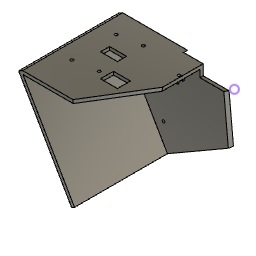
case v32 (Autodesk Fusion 360 design; units mm, degrees)
Autodesk Fusion 360 part; units mm, degrees
note: some values were not read from the file. Set by a fixed rule: which face or edge a step refers to.
ref_plane "WorkPlane2" through (0, 0, 0) normal (0, 0, 1) x (1, 0, 0) in component "Base"
sketch "top" plane through (0, 0, 0) normal (0, 0, 1) x (1, 0, 0) in component "Base"
  line L0 (-48.3808, 27.2591) -> (41.6192, 27.2591)
  line L1 (41.6192, 27.2591) -> (41.6192, -29.7409)
  line L2 (41.6192, -29.7409) -> (-48.3808, -29.7409)
  line L3 (-48.3808, -29.7409) -> (-48.3808, 27.2591)
  line L4 (5.6192, 27.2591) -> (5.6192, -29.7409) construction
  line L5 (5.6192, 27.2591) -> (41.6192, 27.2591)
  line L6 (41.6192, 27.2591) -> (41.6192, 24.2591)
  line L7 (41.6192, 24.2591) -> (5.6192, 24.2591)
  line L8 (5.6192, 24.2591) -> (5.6192, 27.2591)
  dimension "d1" = 90
  dimension "d2" = 57
  dimension "d242" = 54
  dimension "d243" = 3
  constraint horizontal L0
  constraint vertical L1
  constraint horizontal L2
  constraint vertical L3
  constraint coincident L0 L4.start
  constraint coincident L2 L4.end
  constraint perpendicular L2 L4
  constraint horizontal L5
  constraint vertical L6
  constraint horizontal L7
  constraint vertical L8
  constraint coincident L1 L6.end
  measures "d1" distance of L0.start L0.end
  measures "d2" distance of L0.start L2.end
  measures "d242" distance of L3 L4
  measures "d243" distance of L4.start L7.end
ref_plane "WorkPlane1" through (-48.3808, -1.2409, 0) normal (-0.866025, 0, -0.5) x (0, 1, 0) in component "Base"
ref_plane "WorkPlane3" through (0, 0, -1) normal (0, 0, 1) x (1, 0, 0) in component "Base"
sketch "start-dot" plane through (0, 0, -1) normal (0, 0, 1) x (1, 0, 0) in component "Base"
  line L0 (-48.3808, -29.7409) -> (-48.3808, 27.2591)
  line L1 (41.6192, -29.7409) -> (-48.3808, -29.7409)
  line L2 (-4.3808, -30.7409) -> (-14.3808, -30.7409)
  line L3 (-14.3808, -30.7409) -> (-4.3808, -30.7409)
  line L4 (-4.3808, -30.7409) -> (2.6903, -23.6698)
  line L5 (-4.3808, -30.7409) -> (3, -30.7409) construction
  point P0 (-4.3808, -30.7409)
  dimension "d25" = 44
  dimension "d32" = 10
  dimension "d33" = 10
  dimension "d117" = 45
  constraint coincident P0 L2.start
  constraint horizontal L2
  constraint parallel L3 L5
  measures "d25" distance of P0 L0
  measures "d32" distance of P0 L4.end
  measures "d33" distance of P0 L2.end
  measures "d117" angle of L4 L5
ref_plane "WorkPlane3" through (-0.8452, -27.2053, -1) normal (0.696364, -0.696364, 0.173648) x (0.707107, 0.707107, 0) in component "Base"
ref_plane "WorkPlane22" through (-4.3271, -23.7235, -1.8682) normal (0.696364, -0.696364, 0.173648) x (0.707107, 0.707107, 0) in component "Base"
sketch "table-cut" plane through (-48.3808, -1.2409, 0) normal (-0.866025, 0, -0.5) x (0, 1, 0) in component "Base"
  line L0 (-250, -250) -> (250, -250)
  line L1 (250, -250) -> (250, 250)
  line L2 (250, 250) -> (-250, 250)
  line L3 (-250, 250) -> (-250, -250)
  line L4 (-250, -250) -> (250, 250) construction
  line L5 (-250, 250) -> (250, -250) construction
  dimension "d39" = 500
  dimension "d40" = 500
  constraint horizontal L0
  constraint vertical L1
  constraint horizontal L2
  constraint vertical L3
  constraint midpoint origin L5
  measures "d39" distance of L0.start L0.end
  measures "d40" distance of L0.start L2.end
sketch "left-cut" plane through (0, 0, 0) normal (0, 0, 1) x (1, 0, 0) in component "Base"
  line L0 (-250, 250) -> (250, 250)
  line L1 (250, 250) -> (250, -250)
  line L2 (250, -250) -> (-250, -250)
  line L3 (-250, -250) -> (-250, 250)
  line L4 (250, -250) -> (-250, 250) construction
  line L5 (250, 250) -> (-250, -250) construction
  dimension "d41" = 500
  dimension "d42" = 500
  constraint horizontal L0
  constraint vertical L1
  constraint horizontal L2
  constraint vertical L3
  constraint midpoint L4 origin
  measures "d41" distance of L1 L3
  measures "d42" distance of L0.start L2.end
ref_plane "WorkPlane5" through (-3.3808, -29.7409, 0) normal (0, 1, 0) x (-1, 0, 0) in component "Base"
ref_plane "WorkPlane6" through (-3.3808, -49.7409, 0) normal (0, 1, 0) x (-1, 0, 0) in component "Base"
sketch "front-cut" plane through (-3.3808, -49.7409, 0) normal (0, 1, 0) x (1, 0, 0) in component "Base"
  line L0 (-250, -250) -> (250, -250)
  line L1 (250, -250) -> (250, 250)
  line L2 (250, 250) -> (-250, 250)
  line L3 (-250, 250) -> (-250, -250)
  line L4 (250, 250) -> (-250, -250) construction
  line L5 (250, -250) -> (-250, 250) construction
  dimension "d45" = 500
  dimension "d46" = 500
  constraint horizontal L0
  constraint vertical L1
  constraint horizontal L2
  constraint vertical L3
  constraint midpoint origin L4
  measures "d45" distance of L0.start L0.end
  measures "d46" distance of L0.start L2.end
extrude "Extrude1" add sketch "front-cut" along normal blind 500 makes body 1 in component "Base"
extrude "Extrude2" cut sketch "left-cut" against normal blind 500 keep common part bodies 1 in component "Base"
extrude "Extrude3" cut sketch "table-cut" against normal blind 500 keep common part bodies 1 in component "Base"
ref_plane "WorkPlane12" through (-3.3808, 27.2591, 0) normal (0, 1, 0) x (-1, 0, 0) in component "Base"
sketch "back-cut" plane through (-3.3808, 27.2591, 0) normal (0, 1, 0) x (1, 0, 0) in component "Base"
  line L0 (-250, -250) -> (250, -250)
  line L1 (250, -250) -> (250, 250)
  line L2 (250, 250) -> (-250, 250)
  line L3 (-250, 250) -> (-250, -250)
  line L4 (250, 250) -> (-250, -250) construction
  line L5 (250, -250) -> (-250, 250) construction
  dimension "d54" = 500
  dimension "d55" = 500
  constraint horizontal L0
  constraint vertical L1
  constraint horizontal L2
  constraint vertical L3
  constraint midpoint origin L5
  measures "d54" distance of L0.start L0.end
  measures "d55" distance of L0.start L2.end
extrude "Extrude4" cut sketch "back-cut" against normal blind 500 keep common part bodies 1 in component "Base"
ref_plane "WorkPlane10" through (-48.3808, -1.2409, 0) normal (-0.5, 0, 0.866025) x (0, 1, 0) in component "Base"
sketch "thumb-cut" plane through (-4.3271, -23.7235, -1.8682) normal (0.696364, -0.696364, 0.173648) x (0.708719, 0.705362, -0.013464) in component "Base"
  line L0 (250, -250) -> (-250, -250)
  line L1 (-250, -250) -> (-250, 250)
  line L2 (-250, 250) -> (250, 250)
  line L3 (250, 250) -> (250, -250)
  line L4 (250, -250) -> (-250, 250) construction
  line L5 (-250, -250) -> (250, 250) construction
  dimension "d124" = 500
  dimension "d125" = 500
  dimension "d126" = 500
  constraint horizontal L0
  constraint perpendicular L0 L1
  constraint parallel L0 L2
  constraint parallel L1 L3
  constraint coincident L4 origin
  constraint coincident L5 origin
  measures "d124" distance of L0.start L2.end
  measures "d125" distance of L0.end L1.end
  measures "d126" distance of L1.end L2.end
sketch "thumb" plane through (-0.8452, -27.2053, -1) normal (0.696364, -0.696364, 0.173648) x (0.708719, 0.705362, -0.013464) in component "Base"
  line L0 (-4.9995, -0.0684) -> (-22.4426, -47.9927)
  line L1 (-22.4426, -47.9927) -> (11.3864, -60.3054)
  line L2 (11.3864, -60.3054) -> (28.8294, -12.3811)
  line L3 (28.8294, -12.3811) -> (-4.9995, -0.0684)
  line L4 (0, 0) -> (64, 0) construction
  point P0 (-4.9995, -0.0684)
  dimension "d134" = 36
  dimension "d135" = 51
  dimension "d137" = 20
  constraint perpendicular L0 L1
  constraint parallel L0 L2
  constraint parallel L1 L3
  constraint coincident P0 L0.start
  constraint coincident L4.start origin
  constraint horizontal L4
  measures "d134" distance of P0 L2.end
  measures "d135" distance of P0 L0.end
  measures "d137" angle of L3 L4
sketch "zig-zeg-cutout" plane through (-48.3808, -1.2409, 0) normal (-0.866025, 0, -0.5) x (0, 1, 0) in component "Base"
  line L0 (-63.5, 83.6397) -> (43.5, 83.6397)
  line L1 (28.5, 27) -> (28.5, 45)
  line L2 (28.5, 45) -> (25.5, 45)
  line L3 (25.5, 45) -> (25.5, 27)
  line L4 (25.5, 27) -> (28.5, 27)
  line L5 (25.5, 45) -> (29.0656, 45)
  line L6 (29.0656, 45) -> (29.0656, 83.6397)
  line L7 (29.0656, 83.6397) -> (25.5, 83.6397)
  line L8 (25.5, 83.6397) -> (25.5, 45)
  point P0 (-25.92, 83.6397)
  constraint horizontal L0
  constraint coincident L0 P0
  constraint horizontal L5
  constraint vertical L6
  constraint horizontal L7
  constraint vertical L8
  constraint coincident L0 L6.end
  constraint coincident L2.end L3.start
extrude "Extrude24" cut sketch "zig-zeg-cutout" against normal through all bodies 1 in component "Base"
ref_plane "WorkPlane16" through (-6.5609, -11.2409, -72.4341) normal (-0.5, 0, 0.866025) x (0, 1, 0) in component "Base"
sketch "middle-cut" plane through (-6.5609, -11.2409, -72.4341) normal (-0.5, 0, 0.866025) x (0, 1, 0) in component "Base"
  line L0 (-250, -250) -> (250, -250)
  line L1 (250, -250) -> (250, 250)
  line L2 (250, 250) -> (-250, 250)
  line L3 (-250, 250) -> (-250, -250)
  line L4 (-250, -250) -> (250, 250) construction
  line L5 (250, -250) -> (-250, 250) construction
  dimension "d234" = 500
  dimension "d235" = 500
  constraint horizontal L0
  constraint perpendicular L0 L1
  constraint parallel L0 L2
  constraint parallel L1 L3
  constraint coincident L4 origin
  constraint coincident L5 origin
  measures "d234" distance of L0.start L2.end
  measures "d235" distance of L0.start L0.end
extrude "Extrude21" cut sketch "middle-cut" along normal blind 500 keep common part bodies 1 in component "Base"
ref_plane "WorkPlane18" through (20.9871, -8.51, -13.58) normal (0.849684, -0.520984, 0.081324) x (0.522715, 0.852507, 0) in component "Base"
sketch "3pint-cut" plane through (20.9871, -8.51, -13.58) normal (0.849684, -0.520984, 0.081324) x (0.527291, 0.839051, -0.134008) in component "Base"
  line L0 (250, 250) -> (-250, 250)
  line L1 (-250, 250) -> (-250, -250)
  line L2 (-250, -250) -> (250, -250)
  line L3 (250, -250) -> (250, 250)
  line L4 (250, 250) -> (-250, -250) construction
  line L5 (-250, 250) -> (250, -250) construction
  dimension "d238" = 500
  dimension "d239" = 500
  constraint horizontal L0
  constraint perpendicular L0 L1
  constraint parallel L0 L2
  constraint parallel L1 L3
  constraint coincident L4 origin
  constraint coincident L5 origin
  measures "d238" distance of L1.end L2.end
  measures "d239" distance of L0.end L1.end
extrude "Extrude22" cut sketch "3pint-cut" against normal blind 500 keep common part bodies 1 in component "Base"
ref_plane "WorkPlane20" through (-47.3808, -1.2409, -1.7321) normal (-0.5, 0, 0.866025) x (0, 1, 0) in component "Base"
sketch "pinky-cut" plane through (-47.3808, -1.2409, -1.7321) normal (-0.5, 0, 0.866025) x (0, 1, 0) in component "Base"
  line L0 (250, 250) -> (-250, 250)
  line L1 (-250, 250) -> (-250, -250)
  line L2 (-250, -250) -> (250, -250)
  line L3 (250, -250) -> (250, 250)
  line L4 (250, 250) -> (-250, -250) construction
  line L5 (-250, 250) -> (250, -250) construction
  dimension "d257" = 500
  dimension "d258" = 500
  constraint horizontal L0
  constraint perpendicular L0 L1
  constraint parallel L0 L2
  constraint parallel L1 L3
  constraint coincident L4 origin
  constraint coincident L5 origin
  measures "d257" distance of L1.end L2.end
  measures "d258" distance of L0.end L1.end
extrude "Extrude26" cut sketch "pinky-cut" against normal blind 500 keep common part bodies 1 in component "Base"
ref_plane "WorkPlane21" through (0, 0, -8) normal (0, 0, 1) x (1, 0, 0) in component "Base"
sketch "Sketch25" plane through (0, 0, -8) normal (0, 0, 1) x (1, 0, 0) in component "Base"
  point P0 (41.6192, 27.2591)
sketch "left_case" plane through (0, 0, 0) normal (0, 0, 1) x (1, 0, 0) in component "left"
  arc A0 (12.49, 2.5) -> (11, 1.01) centre (12.49, 1.01) ccw
  line L0 (14.5, 32) -> (14.5, 25)
  circle A1 centre (27, 45.5) radius 1.1
  arc A2 (47, 61.01) -> (45.51, 62.5) centre (45.51, 61.01) ccw
  line L1 (45.5, 7) -> (45.5, 17)
  arc A3 (23.51, 59.5) -> (25, 60.99) centre (23.51, 60.99) ccw
  line L2 (62, 56.5) -> (62, 18)
  line L3 (32.5, 17) -> (32.5, 7)
  line L4 (62, 18) -> (83, 18)
  line L5 (47, 57.99) -> (47, 61.01)
  arc A4 (81.51, 2.5) -> (83, 3.99) centre (81.51, 3.99) ccw
  arc A5 (-7, -7.01) -> (-5.51, -8.5) centre (-5.51, -7.01) ccw
  arc A6 (26.49, 62.5) -> (25, 61.01) centre (26.49, 61.01) ccw
  line L6 (27.5, 32) -> (14.5, 32)
  line L7 (14.5, 25) -> (27.5, 25)
  line L8 (45.5, 17) -> (32.5, 17)
  circle A7 centre (27, 11.5) radius 1.1
  line L9 (32.5, 7) -> (45.5, 7)
  arc A8 (47, 57.99) -> (48.49, 56.5) centre (48.49, 57.99) ccw
  line L10 (45.51, 62.5) -> (26.49, 62.5)
  circle A9 centre (9, 42.5) radius 1.1
  circle A10 centre (9, 8.5) radius 1.1
  line L11 (-5.51, 59.5) -> (23.51, 59.5)
  arc A11 (9.51, -8.5) -> (11, -7.01) centre (9.51, -7.01) ccw
  arc A12 (-5.51, 59.5) -> (-7, 58.01) centre (-5.51, 58.01) ccw
  line L12 (12.49, 2.5) -> (81.51, 2.5)
  line L13 (11, -7.01) -> (11, 1.01)
  line L14 (27.5, 25) -> (27.5, 32)
  line L15 (62, 56.5) -> (48.49, 56.5)
  line L16 (-7, -7.01) -> (-7, 58.01)
  line L17 (83, 3.99) -> (83, 18)
  line L18 (-5.51, -8.5) -> (9.51, -8.5)
  line L19 (25, 61.01) -> (25, 60.99)
  circle A13 centre (63, 14) radius 1.1
  circle A14 centre (60.5, 39.5) radius 1.1
  line L20 (62, 18) -> (90.5, 18)
  line L21 (90.5, 18) -> (90.5, 64.5)
  line L22 (90.5, 64.5) -> (62, 64.5)
  line L23 (62, 64.5) -> (62, 18)
  constraint horizontal L20
  constraint vertical L21
  constraint horizontal L22
  constraint vertical L23
sketch "left_pcb_edgecut" plane through (0, 0, 0) normal (0, 0, 1) x (1, 0, 0) in component "left"
  arc A0 (-5.51, 59.5) -> (-7, 58.01) centre (-5.51, 58.01) ccw
  line L0 (45.51, 62.5) -> (26.49, 62.5)
  line L1 (47, 57.99) -> (47, 61.01)
  line L2 (12.49, 2.5) -> (81.51, 2.5)
  arc A1 (23.51, 59.5) -> (25, 60.99) centre (23.51, 60.99) ccw
  arc A2 (-7, -7.01) -> (-5.51, -8.5) centre (-5.51, -7.01) ccw
  arc A3 (47, 57.99) -> (48.49, 56.5) centre (48.49, 57.99) ccw
  arc A4 (26.49, 62.5) -> (25, 61.01) centre (26.49, 61.01) ccw
  line L3 (25, 61.01) -> (25, 60.99)
  line L4 (-7, -7.01) -> (-7, 58.01)
  line L5 (-5.51, -8.5) -> (9.51, -8.5)
  arc A5 (9.51, -8.5) -> (11, -7.01) centre (9.51, -7.01) ccw
  arc A6 (83, 52.01) -> (81.51, 53.5) centre (81.51, 52.01) ccw
  arc A7 (81.51, 2.5) -> (83, 3.99) centre (81.51, 3.99) ccw
  line L6 (83, 3.99) -> (83, 52.01)
  line L7 (63.51, 56.5) -> (48.49, 56.5)
  arc A8 (65, 55.01) -> (63.51, 56.5) centre (63.51, 55.01) ccw
  line L8 (81.51, 53.5) -> (66.49, 53.5)
  line L9 (65, 54.99) -> (65, 55.01)
  arc A9 (65, 54.99) -> (66.49, 53.5) centre (66.49, 54.99) ccw
  line L10 (11, -7.01) -> (11, 1.01)
  arc A10 (47, 61.01) -> (45.51, 62.5) centre (45.51, 61.01) ccw
  line L11 (-5.51, 59.5) -> (23.51, 59.5)
  arc A11 (12.49, 2.5) -> (11, 1.01) centre (12.49, 1.01) ccw
extrude "Extrude3'" add sketch "left_pcb_edgecut" along normal blind 3.6 separate body makes body 2 in component "left"
sketch "thumb_case (1)" plane through (0, 0, 0) normal (0, 0, 1) x (1, 0, 0) in component "thumb"
  arc A0 (27, 41) -> (25.5, 42.5) centre (25.5, 41) ccw
  circle A1 centre (9, 34) radius 1.1
  line L0 (-9, -7) -> (-9, 41)
  arc A2 (25.5, -8.5) -> (27, -7) centre (25.5, -7) ccw
  circle A3 centre (9, 0) radius 1.1
  line L1 (20, 6) -> (20, 28)
  line L2 (-7.5, 42.5) -> (25.5, 42.5)
  line L3 (9, 6) -> (20, 6)
  arc A4 (-9, -7) -> (-7.5, -8.5) centre (-7.5, -7) ccw
  line L4 (9, 28) -> (9, 6)
  arc A5 (-7.5, 42.5) -> (-9, 41) centre (-7.5, 41) ccw
  line L5 (20, 28) -> (9, 28)
  line L6 (-7.5, -8.5) -> (25.5, -8.5)
  line L7 (27, -7) -> (27, 41)
extrude "Extrude3''" add sketch "thumb_case (1)" along normal blind 3.6 separate body contours A0 L0 A2 L2 A4 A5 L6 L7 | L1 L3 L4 L5 makes body 3 in component "thumb"
extrude "Extrude4'" add sketch "thumb_case (1)" along normal blind 11 from surface at 3.6 separate body contours A0 L0 A2 L2 A4 A5 L6 L7 | A1 | A3 | L1 L3 L4 L5 makes body 4 in component "thumb"
extrude "Extrude2'" add sketch "left_pcb_edgecut" along normal blind 11 from surface at 3.6 separate body sketch seen with x (1, 0, 0) y (0, 1, 0) z (0, 0, 1) at (-41.3808, -32.2409, 0) makes body 5
copy_body "CutPasteBodies1" bodies 5 body 5 seen with x (1, 0, 0) y (0, 1, 0) z (0, 0, 1) at (41.3808, 32.2409, 0) removing the originals makes body 6 in component "left"
sketch "left_screw" plane through (0, 0, 0) normal (0, 0, 1) x (1, 0, 0) in component "left"
  arc A0 (83, 52.01) -> (81.51, 53.5) centre (81.51, 52.01) ccw
  line L0 (24.5, 48) -> (24.5, 43)
  arc A1 (26.49, 62.5) -> (25, 61.01) centre (26.49, 61.01) ccw
  line L1 (61.45, 12.45) -> (64.55, 12.45)
  line L2 (-5.51, 59.5) -> (23.51, 59.5)
  circle A2 centre (63, 14) radius 1.1
  line L3 (6.5, 45) -> (6.5, 40)
  line L4 (61.45, 15.55) -> (61.45, 12.45)
  circle A3 centre (27, 11.5) radius 1.1
  line L5 (7.45, 10.05) -> (7.45, 6.95)
  arc A4 (23.51, 59.5) -> (25, 60.99) centre (23.51, 60.99) ccw
  line L6 (10.55, 6.95) -> (10.55, 10.05)
  circle A5 centre (9, 8.5) radius 1.1
  line L7 (65.5, 11.5) -> (65.5, 16.5)
  line L8 (58, 42) -> (58, 37)
  line L9 (58, 37) -> (63, 37)
  line L10 (10.55, 40.95) -> (10.55, 44.05)
  line L11 (62.05, 37.95) -> (62.05, 41.05)
  line L12 (10.55, 10.05) -> (7.45, 10.05)
  line L13 (29.5, 43) -> (29.5, 48)
  line L14 (25, 61.01) -> (25, 60.99)
  arc A6 (65, 55.01) -> (63.51, 56.5) centre (63.51, 55.01) ccw
  circle A7 centre (27, 45.5) radius 1.1
  arc A8 (9.51, -8.5) -> (11, -7.01) centre (9.51, -7.01) ccw
  line L15 (63.51, 56.5) -> (48.49, 56.5)
  circle A9 centre (60.5, 39.5) radius 1.1
  circle A10 centre (9, 42.5) radius 1.1
  line L16 (11.5, 6) -> (11.5, 11)
  line L17 (45.51, 62.5) -> (26.49, 62.5)
  line L18 (-5.51, -8.5) -> (9.51, -8.5)
  line L19 (11, -7.01) -> (11, 1.01)
  line L20 (29.5, 9) -> (29.5, 14)
  line L21 (25.45, 43.95) -> (28.55, 43.95)
  line L22 (6.5, 11) -> (6.5, 6)
  line L23 (62.05, 41.05) -> (58.95, 41.05)
  line L24 (28.55, 47.05) -> (25.45, 47.05)
  line L25 (7.45, 44.05) -> (7.45, 40.95)
  arc A11 (12.49, 2.5) -> (11, 1.01) centre (12.49, 1.01) ccw
  line L26 (28.55, 43.95) -> (28.55, 47.05)
  line L27 (25.45, 13.05) -> (25.45, 9.95)
  line L28 (60.5, 16.5) -> (60.5, 11.5)
  line L29 (24.5, 9) -> (29.5, 9)
  line L30 (64.55, 12.45) -> (64.55, 15.55)
  line L31 (24.5, 14) -> (24.5, 9)
  line L32 (11.5, 11) -> (6.5, 11)
  line L33 (11.5, 40) -> (11.5, 45)
  line L34 (10.55, 44.05) -> (7.45, 44.05)
  line L35 (7.45, 40.95) -> (10.55, 40.95)
  arc A12 (65, 54.99) -> (66.49, 53.5) centre (66.49, 54.99) ccw
  line L36 (25.45, 9.95) -> (28.55, 9.95)
  line L37 (6.5, 6) -> (11.5, 6)
  line L38 (28.55, 13.05) -> (25.45, 13.05)
  line L39 (28.55, 9.95) -> (28.55, 13.05)
  arc A13 (47, 57.99) -> (48.49, 56.5) centre (48.49, 57.99) ccw
  line L40 (25.45, 47.05) -> (25.45, 43.95)
  line L41 (24.5, 43) -> (29.5, 43)
  line L42 (11.5, 45) -> (6.5, 45)
  line L43 (63, 37) -> (63, 42)
  line L44 (63, 42) -> (58, 42)
  line L45 (12.49, 2.5) -> (81.51, 2.5)
  arc A14 (81.51, 2.5) -> (83, 3.99) centre (81.51, 3.99) ccw
  arc A15 (-7, -7.01) -> (-5.51, -8.5) centre (-5.51, -7.01) ccw
  line L46 (-7, -7.01) -> (-7, 58.01)
  arc A16 (-5.51, 59.5) -> (-7, 58.01) centre (-5.51, 58.01) ccw
  arc A17 (47, 61.01) -> (45.51, 62.5) centre (45.51, 61.01) ccw
  line L47 (29.5, 14) -> (24.5, 14)
  line L48 (6.5, 40) -> (11.5, 40)
  line L49 (65.5, 16.5) -> (60.5, 16.5)
  line L50 (60.5, 11.5) -> (65.5, 11.5)
  line L51 (29.5, 48) -> (24.5, 48)
  line L52 (47, 57.99) -> (47, 61.01)
  line L53 (64.55, 15.55) -> (61.45, 15.55)
  line L54 (58.95, 37.95) -> (62.05, 37.95)
  line L55 (65, 54.99) -> (65, 55.01)
  line L56 (81.51, 53.5) -> (66.49, 53.5)
  line L57 (83, 3.99) -> (83, 52.01)
  line L58 (7.45, 6.95) -> (10.55, 6.95)
  line L59 (58.95, 41.05) -> (58.95, 37.95)
sketch "thumb_screw" plane through (0, 0, 0) normal (0, 0, 1) x (1, 0, 0) in component "thumb"
  line L0 (10.55, 32.45) -> (10.55, 35.55)
  line L1 (-7.5, 42.5) -> (25.5, 42.5)
  arc A0 (-7.5, 42.5) -> (-9, 41) centre (-7.5, 41) ccw
  line L2 (11.5, -2.5) -> (11.5, 2.5)
  circle A1 centre (9, 0) radius 1.1
  arc A2 (25.5, -8.5) -> (27, -7) centre (25.5, -7) ccw
  circle A3 centre (9, 34) radius 1.1
  line L3 (10.55, 1.55) -> (7.45, 1.55)
  arc A4 (27, 41) -> (25.5, 42.5) centre (25.5, 41) ccw
  line L4 (27, -7) -> (27, 41)
  line L5 (6.5, -2.5) -> (11.5, -2.5)
  line L6 (7.45, 32.45) -> (10.55, 32.45)
  line L7 (7.45, 35.55) -> (7.45, 32.45)
  arc A5 (-9, -7) -> (-7.5, -8.5) centre (-7.5, -7) ccw
  line L8 (7.45, -1.55) -> (10.55, -1.55)
  line L9 (6.5, 36.5) -> (6.5, 31.5)
  line L10 (-7.5, -8.5) -> (25.5, -8.5)
  line L11 (10.55, -1.55) -> (10.55, 1.55)
  line L12 (-9, -7) -> (-9, 41)
  line L13 (10.55, 35.55) -> (7.45, 35.55)
  line L14 (11.5, 31.5) -> (11.5, 36.5)
  line L15 (6.5, 31.5) -> (11.5, 31.5)
  line L16 (11.5, 36.5) -> (6.5, 36.5)
  line L17 (11.5, 2.5) -> (6.5, 2.5)
  line L18 (6.5, 2.5) -> (6.5, -2.5)
  line L19 (7.45, 1.55) -> (7.45, -1.55)
shell "Shell3" thickness 2.5 removed faces 3 at (12.7625, -0.4075, -61.2778) at (13.085, -25.0742, -37.133) at (-18.845, -49.7409, -24.1447) on bodies 1 in component "Base"
sketch "thumb-holder" plane through (-0.8452, -27.2053, -1) normal (0.696364, -0.696364, 0.173648) x (0.707107, 0.707107, 0) in component "Base"
  line L0 (-23.0966, -47.6814) -> (10.5608, -60.4554)
  line L1 (10.5608, -60.4554) -> (28.6574, -12.7741)
  line L2 (28.6574, -12.7741) -> (-5, 0)
  line L3 (-5, 0) -> (-23.0966, -47.6814)
  line L4 (-22.5644, -46.279) -> (-5.5323, -1.4024)
  line L5 (-5, 0) -> (10.5608, -60.4554) construction
  line L6 (-23.0966, -47.6814) -> (28.6574, -12.7741) construction
  line L7 (-12.0001, -35.4299) -> (-13.7743, -40.1046)
  line L8 (-13.7743, -40.1046) -> (-9.0996, -41.8788)
  line L9 (-9.0996, -41.8788) -> (-7.3254, -37.2041)
  line L10 (-7.3254, -37.2041) -> (-12.0001, -35.4299)
  line L11 (-4.6648, -16.5643) -> (0.0098, -18.3385)
  line L12 (0.0098, -18.3385) -> (1.784, -13.6638)
  line L13 (1.784, -13.6638) -> (-2.8906, -11.8896)
  line L14 (-2.8906, -11.8896) -> (-4.6648, -16.5643)
  line L15 (18.9206, -19.2558) -> (14.246, -17.4816)
  line L16 (14.246, -17.4816) -> (12.4718, -22.1562)
  line L17 (12.4718, -22.1562) -> (17.1465, -23.9304)
  line L18 (17.1465, -23.9304) -> (18.9206, -19.2558)
  line L19 (9.4504, -44.5999) -> (4.7758, -42.8257)
  line L20 (4.7758, -42.8257) -> (3.0016, -47.5004)
  line L21 (3.0016, -47.5004) -> (7.6762, -49.2746)
  line L22 (7.6762, -49.2746) -> (9.4504, -44.5999)
  dimension "d325" = 5
  dimension "d326" = 5
  dimension "d327" = 5
  dimension "d328" = 5
  dimension "d329" = 5
  dimension "d330" = 5
  dimension "d331" = 5
  dimension "d332" = 5
  constraint coincident L1.end L2.start
  constraint coincident L2.end L3.start
  constraint coincident L0.end L1.start
  constraint coincident L0.start L3.end
  constraint perpendicular L7 L8
  constraint parallel L7 L9
  constraint parallel L8 L10
  constraint parallel L4 L7
  constraint perpendicular L11 L14
  constraint parallel L12 L14
  constraint parallel L11 L13
  constraint perpendicular L16 L17
  constraint parallel L16 L18
  constraint parallel L15 L17
  constraint perpendicular L20 L21
  constraint parallel L20 L22
  constraint parallel L19 L21
  measures "d325" distance of L7.start L9.end
  measures "d326" distance of L8.end L9.end
  measures "d327" distance of L13.end L12.end
  measures "d328" distance of L11.end L12.end
  measures "d329" distance of L15.end L15.start
  measures "d330" distance of L17.end L15.start
  measures "d331" distance of L19.end L19.start
  measures "d332" distance of L19.start L21.end
extrude "Extrude36" add sketch "thumb-holder" against normal blind 12.5 separate body contours L7 L8 L9 L10 | L11 L12 L13 L14 | L15 L16 L17 L18 | L19 L20 L21 L22 makes body 7 at (8.6413, -11.6068, -24.4794) makes body 8 at (6.557, -25.9554, -49.6671) makes body 9 at (-1.0344, -25.3296, -16.7143) makes body 10 at (-4.5853, -34.6614, -39.897) in component "Base"
extrude "Extrude38" cut sketch "thumb_case (1)" against normal blind 2.5 contours A1 | A3 | L1 L3 L4 L5 sketch seen with x (0.704664, 0.617525, -0.349445) y (0.136109, 0.365705, 0.920725) z (0.696364, -0.696364, 0.173648) at (-3.8234, -40.7256, -43.2758) bodies 7 8 10 9 in component "Base"
extrude "Extrude39" add sketch "thumb_case (1)" against normal blind 2.5 sketch seen with x (0.704664, 0.617525, -0.349445) y (0.136109, 0.365705, 0.920725) z (0.696364, -0.696364, 0.173648) at (-3.8234, -40.7256, -43.2758) bodies 7 8 9 10 in component "Base"
extrude "Extrude40" cut sketch "left_case" against normal blind 2.5 contours L0 L6 L7 L14 | A1 | L1 L3 L8 L9 | A7 | A9 | A10 | A13 | A14 sketch seen with x (1, 0, 0) y (0, 1, 0) z (0, 0, 1) at (-41.3808, -32.2409, 0) bodies 1 in component "Base"
extrude "Extrude41" add sketch "left_screw" against normal blind 4 contours L0 L13 L41 L51 | L3 L33 L42 L48 | L8 L9 L43 L44 | L16 L22 L32 L37 | L20 L29 L31 L47 sketch seen with x (1, 0, 0) y (0, 1, 0) z (0, 0, 1) at (-41.3808, -32.2409, 0) bodies 1 in component "Base"
extrude "Extrude16" cut sketch "left_case" against normal blind 8 contours L2 L4 L20 L21 L22 L23 sketch seen with x (1, 0, 0) y (0, 1, 0) z (0, 0, 1) at (-41.3808, -32.2409, 0) bodies 1 in component "Base"
sketch "rubber-feet" plane through (-48.3808, -1.2409, 0) normal (-0.866025, 0, -0.5) x (0, 1, 0) in component "Base"
  circle A0 centre (-42.5, 77.6397) radius 4.5
  line L0 (-48.5, 83.6397) -> (-48.5, 2)
  line L1 (-48.5, 83.6397) -> (25.5, 83.6397)
  circle A1 centre (-42.5, 8) radius 4.5
  circle A2 centre (19.5, 77.6397) radius 4.5
  circle A3 centre (22.5, 8) radius 4.5
  line L2 (25.5, 27) -> (25.5, 83.6397)
  line L3 (28.5, 2) -> (-48.5, 2)
  line L4 (28.5, 27) -> (28.5, 2)
  line L5 (-20, 4.5) -> (-46, 4.5)
  line L6 (-46, 4.5) -> (-46, 81.1397)
  line L7 (-46, 81.1397) -> (-20, 81.1397)
  line L8 (-20, 81.1397) -> (-20, 4.5)
  circle A4 centre (-42.5, 8) radius 5.5
  circle A5 centre (-42.5, 77.6397) radius 5.5
  dimension "d367" = 9
  dimension "d368" = 6
  dimension "d369" = 6
  dimension "d370" = 9
  dimension "d371" = 9
  dimension "d372" = 9
  dimension "d373" = 6
  dimension "d374" = 6
  dimension "d375" = 6
  dimension "d376" = 6
  dimension "d377" = 6
  dimension "d378" = 6
  dimension "d381" = 26
  dimension "d382" = 2.5
  dimension "d383" = 2.5
  dimension "d384" = 2.5
  dimension "d385" = 11
  dimension "d386" = 11
  constraint horizontal L5
  constraint vertical L6
  constraint horizontal L7
  constraint vertical L8
  constraint concentric A1 A4
  constraint concentric A0 A5
  measures "d367" diameter of A0
  measures "d368" distance of A0.centre L0
  measures "d369" distance of A0.centre L1
  measures "d370" diameter of A1
  measures "d371" diameter of A2
  measures "d372" diameter of A3
  measures "d373" distance of A2.centre L2
  measures "d374" distance of L1 A2.centre
  measures "d375" distance of A3.centre L3
  measures "d376" distance of A3.centre L4
  measures "d377" distance of A1.centre L3
  measures "d378" distance of L0 A1.centre
  measures "d381" distance of L6 L8
  measures "d382" distance of L1 L7
  measures "d383" distance of L3 L5
  measures "d384" distance of L0 L6
  measures "d385" diameter of A4
  measures "d386" diameter of A5
extrude "Extrude44" cut sketch "rubber-feet" against normal blind 1.5 contours A0 L6 L7 | A0 L7 | A0 L6 | A1 L6 | A1 L5 L6 | A1 L5 | A2 | A3 picked at (-43.659, 78.7339) picked at (-43.2475, 8.5869) bodies 1 in component "Base"
extrude "Extrude45" cut sketch "rubber-feet" against normal blind 0.8 contours L5 L6 L7 L8 A4 A5 bodies 1 in component "Base"
move_face "OffsetFaces1" offset 3 1 faces at (-27.1292, 24.7591, -8.3225) on bodies 1 in component "Base"
sketch "mount-holes" plane through (-3.3808, 27.2591, 0) normal (0, 1, 0) x (1, 0, 0) in component "Base"
  circle A0 centre (-3.9668, 51.0716) radius 1
  circle A1 centre (-13.9668, 33.7511) radius 1
  line L0 (-31.5, 23.3827) -> (-3.1801, 72.4341)
  dimension "d396" = 2
  dimension "d397" = 2
  dimension "d398" = 10
  dimension "d399" = 10
  dimension "d400" = 20
  measures "d396" diameter of A0
  measures "d397" diameter of A1
  measures "d398" distance of A1.centre L0
  measures "d399" distance of A0.centre L0
  measures "d400" distance of A0.centre A1.centre
extrude "Extrude47" cut sketch "mount-holes" against normal blind 8 bodies 1 in component "Base"
ref_plane "WorkPlane15" through (26.6192, -1.2409, -129.9038) normal (-0.5, 0, 0.866025) x (0, 1, 0) in component "Base"
mirror "Mirror1" [suppressed] in component "Base"
mirror "Mirror2" [suppressed] in component "Base"
component "left" placed x (1, 0, 0) y (0, 1, 0) z (0, 0, 1) at (-41.3808, -32.2409, 0)
component "Base" placed x (1, 0, 0) y (0, 1, 0) z (0, 0, 1) at (0, 0, 0)
component "thumb" placed x (0.704664, 0.617525, -0.349445) y (0.136109, 0.365705, 0.920725) z (0.696364, -0.696364, 0.173648) at (-3.8234, -40.7256, -43.2758)
hidden bodies 7
equation "angleA = 45 deg"
equation "angleB = 10 deg"
equation "d24 = -dd3"
equation "d25 = dd1"
equation "d26 = dd2"
equation "d31 = 90 deg - angleB"
equation "angleC = 20 deg"
equation "lagre = 50 cm"
equation "d39 = lagre"
equation "d40 = d39"
equation "d41 = lagre"
equation "d42 = d41"
equation "d45 = lagre"
equation "d46 = d45"
equation "d47 = lagre"
equation "d49 = -lagre"
equation "d51 = -lagre"
equation "d54 = lagre"
equation "d55 = lagre"
equation "d56 = -lagre"
equation "dd1 = 44 mm"
equation "dd2 = 1 mm"
equation "dd3 = 1 mm"
equation "pcb_with_hot_swap = 3.6 mm"
equation "d117 = angleA"
equation "d124 = lagre"
equation "d126 = lagre"
equation "d136 = dd2"
equation "d137 = angleC"
equation "nn_depth_from_pcb = 8 mm"
equation "d180 = -nn_depth_from_pcb"
equation "d186 = pcb_with_hot_swap"
equation "d188 = pcb_with_hot_swap"
equation "d190 = pcb_with_hot_swap"
equation "d207 = pcb_with_hot_swap"
equation "d234 = lagre"
equation "d235 = lagre"
equation "d236 = lagre"
equation "d238 = lagre"
equation "d239 = lagre"
equation "d240 = -lagre"
equation "d257 = lagre"
equation "d258 = lagre"
equation "d259 = -lagre"
equation "d291 = -nn_depth_from_pcb"
equation "caseThikness = 2.5 mm"
equation "screwBump = 1.5 mm"
equation "d333 = -caseThikness - 10 mm"
equation "d337 = -caseThikness"
equation "d344 = -caseThikness"
equation "d348 = -caseThikness"
equation "d350 = -caseThikness - screwBump"
equation "d364 = caseThikness"
equation "d369 = d368"
equation "d373 = d368"
equation "d374 = d368"
equation "d375 = d377"
equation "d376 = d377"
equation "d377 = d368"
equation "d378 = d368"
equation "d382 = caseThikness"
equation "d383 = caseThikness"
equation "d384 = caseThikness"
equation "d399 = d398"
